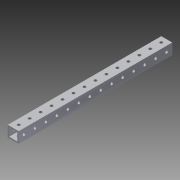
# Autodesk Inventor part: Chassis Part10 (26x28)
Saved by Autodesk Inventor 2013 (Build 170138000, 138)
## iProperties
Created: 2013-01-18
Part Number: Chassis Part10 (26x28)
Material: Aluminum 6061
Document SubType Name: Modeling
Designer: Moses
Mass: 255.5 g
Surface Area: 636.426 cm^2
Volume: 94.2805 cm^3
Density: 2.71 g/cm^3
Author: Moses
Autodesk Inventor part; units mm, degrees
ref_plane "YZ Plane" through (0, 0, 0) normal (1, 0, 0) x (0, 1, 0)
ref_plane "XZ Plane" through (0, 0, 0) normal (0, 1, 0) x (-1, 0, 0)
ref_plane "XY Plane" through (0, 0, 0) normal (0, 0, 1) x (1, 0, 0)
sketch "Sketch1" plane through (0, 0, 0) normal (0, 0, 1) x (1, 0, 0)
  line L0 (0, 0) -> (25.4, 0)
  line L1 (25.4, 0) -> (25.4, 25.4)
  line L2 (25.4, 25.4) -> (0, 25.4)
  line L3 (0, 25.4) -> (0, 0)
  line L4 (3.175, 22.225) -> (22.225, 22.225)
  line L5 (22.225, 22.225) -> (22.225, 3.175)
  line L6 (22.225, 3.175) -> (3.175, 3.175)
  line L7 (3.175, 3.175) -> (3.175, 22.225)
  dimension "d0" = 25.4
  dimension "d1" = 25.4
  dimension "d2" = 3.175
  constraints: 16 end point, 4 parallel, 2 perpendicular, 1 horizontal, 3 other
  measures "d0" distance of L2.end L1.end
  measures "d1" distance of L1.end L0.end
  measures "d2" distance between parallel lines of L1 L5
extrude "Extrusion1" add sketch "Sketch1" along normal blind 355.6
sketch "Sketch2" plane through (25.4, 0, 0) normal (1, 0, 0) x (0, 0, -1)
  line L0 (-355.6, 0) -> (-355.6, 25.4) projected
  line L1 (0, 0) -> (-355.6, 0) projected
  line L2 (-355.6, 12.7) -> (-342.9, 12.7) construction
  circle A0 centre (-342.9, 12.7) radius 3.302 construction
  circle A1 centre (-317.5, 12.7) radius 3.302
  circle A2 centre (-292.1, 12.7) radius 3.302
  circle A3 centre (-266.7, 12.7) radius 3.302
  circle A4 centre (-241.3, 12.7) radius 3.302
  circle A5 centre (-215.9, 12.7) radius 3.302
  circle A6 centre (-190.5, 12.7) radius 3.302
  circle A7 centre (-165.1, 12.7) radius 3.302
  circle A8 centre (-139.7, 12.7) radius 3.302
  circle A9 centre (-114.3, 12.7) radius 3.302
  circle A10 centre (-88.9, 12.7) radius 3.302
  circle A11 centre (-63.5, 12.7) radius 3.302
  circle A12 centre (-38.1, 12.7) radius 3.302
  circle A13 centre (-12.7, 12.7) radius 3.302
  line L3 (0, 0) -> (0, 25.4) projected
  circle A14 centre (-342.9, 12.7) radius 3.302
  circle A15 centre (-12.7, 12.7) radius 3.302
  line L4 (-12.7, 12.7) -> (0, 12.7) construction
  dimension "d5" = 12.7
  dimension "d7" = 6.604
  dimension "d10" = 355.6
  dimension "d13" = 25.4
  dimension "d19" = 12.7
  dimension "d20" = 6.604
  dimension "d21" = 6.604
  dimension "d22" = 12.7
  constraints: 16 centre point, 4 end point, 2 horizontal, 2 midpoint, 1 coincident, 1 parallel, 1 point on line, 26 other
  measures "d5" distance of L2.start L2.end
  measures "d7" diameter of A0
  measures "d10" distance of L3.end L0.end
  measures "d13" distance of A0.centre A1.centre
  measures "d19" distance of L4.start L4.end
  measures "d20" diameter of A15
  measures "d21" diameter of A14
  measures "d22" distance from line of L0 A14.centre
extrude "Extrusion2" cut sketch "Sketch2" against normal through all
sketch "Sketch3" plane through (0, 25.4, 0) normal (0, 1, 0) x (1, 0, 0)
  line L0 (25.4, 0) -> (0, 0) projected
  line L1 (25.4, -355.6) -> (0, -355.6) projected
  circle A0 centre (12.7, -342.9) radius 3.302
  line L2 (12.7, -355.6) -> (12.7, 0) construction
  circle A1 centre (12.7, -317.5) radius 3.302
  circle A2 centre (12.7, -292.1) radius 3.302
  circle A3 centre (12.7, -266.7) radius 3.302
  circle A4 centre (12.7, -241.3) radius 3.302
  circle A5 centre (12.7, -215.9) radius 3.302
  circle A6 centre (12.7, -190.5) radius 3.302
  circle A7 centre (12.7, -165.1) radius 3.302
  circle A8 centre (12.7, -139.7) radius 3.302
  circle A9 centre (12.7, -114.3) radius 3.302
  circle A10 centre (12.7, -88.9) radius 3.302
  circle A11 centre (12.7, -63.5) radius 3.302
  circle A12 centre (12.7, -38.1) radius 3.302
  circle A13 centre (12.7, -12.7) radius 3.302
  dimension "d23" = 6.604
  dimension "d25" = 12.7
  dimension "d28" = 25.4
  constraints: 14 centre point, 2 end point, 2 midpoint, 1 point on line, 1 vertical, 26 other
  measures "d23" diameter of A0
  measures "d25" distance from line of L1 A0.centre
  measures "d28" distance of A0.centre A1.centre
extrude "Extrusion3" cut sketch "Sketch3" against normal blind 25.4
equation "\"d20\" = d7"
equation "\"d21\" = d7"
equation "\"d22\" = d19"
body "Solid1"
